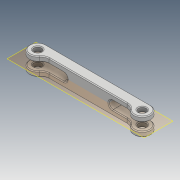
# Autodesk Inventor part: bar_act_ab
Saved by Autodesk Inventor 2018 (Build 220112000, 112)
## iProperties
Created: 2019-01-31
Part Number: bar_act_ab
Material: Generic
Document SubType Name: Modeling
Designer: Tsche
Density: 1 g/cm^3
Appearance: Default
Author: Tsche
Autodesk Inventor part; units mm, degrees
ref_plane "YZ Plane" through (0, 0, 0) normal (1, 0, 0) x (0, 1, 0)
ref_plane "XZ Plane" through (0, 0, 0) normal (0, 1, 0) x (-1, 0, 0)
ref_plane "XY Plane" through (0, 0, 0) normal (0, 0, 1) x (1, 0, 0)
sketch "Sketch1" plane through (0, 0, 0) normal (0, 0, 1) x (1, 0, 0)
  circle A0 centre (20.2406, 0) radius 1.4625
  line L0 (20.2406, 3.25) -> (-2.6872, 3.25)
  line L1 (-446494.9011, 0) -> (446494.9011, 0) construction
  line L2 (0, -0.75) -> (15.1171, -0.75)
  arc A1 (17.6789, -2) -> (20.2406, 3.25) centre (20.2406, 0) ccw
  arc A2 (17.6789, -2) -> (15.1171, -0.75) centre (15.1171, -4) ccw
  line L3 (0, -446500.8256) -> (0, 446500.0254) construction
  circle A3 centre (-20.2406, 0) radius 1.4625
  line L4 (-20.2406, 3.25) -> (-2.6872, 3.25)
  line L5 (446494.9011, 0) -> (-446494.9011, 0) construction
  line L6 (0, -0.75) -> (-15.1171, -0.75)
  arc A4 (-20.2406, 3.25) -> (-17.6789, -2) centre (-20.2406, 0) ccw
  arc A5 (-15.1171, -0.75) -> (-17.6789, -2) centre (-15.1171, -4) ccw
  point P0 (0, 0)
  dimension "d0" = 4
  dimension "d1" = 3.25
  dimension "d2" = 3.25
  dimension "d3" = 2.925
  dimension "d4" = 40.4813
  constraints: 10 end point, 8 horizontal alignment, 8 point on circle, 6 centre point, 3 equal radius, 3 tangent, 2 coincident, 2 horizontal, 2 point on line, 2 other
  measures "d0" distance between parallel lines of L0 L2
  measures "d1" radius of A1
  measures "d2" radius of A2
  measures "d3" diameter of A0
  measures "d4" distance of A0.centre A3.centre
extrude "Extrusion1" add sketch "Sketch1" along normal blind 7
ref_plane "Work Plane1" through (0, 0, 3.5) normal (0, 0, 1) x (1, 0, 0)
sketch "Sketch2" plane through (-20.2406, 3.25, 0) normal (0, 1, 0) x (1, 0, 0)
  line L0 (53.1275, -3.5) -> (-12.6463, -3.5) construction
  line L1 (43.7313, 0) -> (43.7313, -7) construction
  line L2 (43.7313, -1.9625) -> (29.7613, -1.9625)
  line L3 (43.7313, -5.0375) -> (29.7613, -5.0375)
  arc A0 (29.7613, -1.9625) -> (29.7613, -5.0375) centre (29.7613, -3.5) ccw
  line L4 (43.7313, -1.9625) -> (43.7313, -5.0375)
  line L5 (20.2406, 1.4) -> (20.2406, -8.4) construction
  line L6 (-3.25, -1.9625) -> (10.72, -1.9625)
  line L7 (-3.25, -5.0375) -> (10.72, -5.0375)
  arc A1 (10.72, -5.0375) -> (10.72, -1.9625) centre (10.72, -3.5) ccw
  line L8 (-3.25, -1.9625) -> (-3.25, -5.0375)
  point P0 (20.2406, 0)
  dimension "d7" = 3.075
  dimension "d9" = 13.97
  constraints: 12 end point, 7 symmetric about line, 4 point on circle, 2 centre point, 1 collinear, 1 perpendicular, 1 point on line, 1 tangent, 1 other
  measures "d7" distance between parallel lines of L2 L3
  measures "d9" distance from line of L1 A0.centre
extrude "Extrusion2" cut sketch "Sketch2" against normal through all
chamfer "Chamfer1" distance 0.3 angle 45 26 edges at (0, -0.75, 7) (16.5424, -1.0792, 7) (23.1615, -1.4252, 7) (0, 3.25, 7) (-23.1615, -1.4252, 7) (-16.5424, -1.0792, 7) (0, -0.75, 0) (16.5424, -1.0792, 0) (23.1615, -1.4252, 0) (0, 3.25, 0) (-23.1615, -1.4252, 0) (-16.5424, -1.0792, 0) (7.9831, -0.75, 3.5) (12.3189, -0.75, 5.0375) (16.5424, -1.0792, 5.0375) (23.1615, -1.4252, 5.0375) (23.1615, -1.4252, 1.9625) (16.5424, -1.0792, 1.9625) (12.3189, -0.75, 1.9625) (-16.5424, -1.0792, 1.9625) (-23.1615, -1.4252, 1.9625) (-14.8806, 3.25, 1.9625) (-7.9831, 3.25, 3.5) (-14.8806, 3.25, 5.0375) (-23.1615, -1.4252, 5.0375) (-16.5424, -1.0792, 5.0375)
fillet "Fillet1" radius 0.3 8 edges at (-21.7031, 0, 0) (-21.7031, 0, 1.9625) (-21.7031, 0, 5.0375) (-21.7031, 0, 7) (18.7781, 0, 5.0375) (18.7781, 0, 7) (18.7781, 0, 1.9625) (18.7781, 0, 0)
equation "\"d0\" = bar_thickness"
equation "\"d1\" = 0.5 * bar_diameter"
equation "\"d2\" = 0.5 * bar_diameter"
equation "\"d3\" = bore_press"
equation "\"d4\" = bar_act_length_ab"
equation "\"d5\" = bar_width"
equation "\"d7\" = hinge_thickness + finger_link_clearence"
equation "\"d10\" = hinge_thickness"
equation "\"d12\" = champfer"
equation "\"bar_length_bc\" = finger_part_B_length"
equation "\"hinge_thickness\" = 3"
equation "\"bar_diameter\" = 6.5"
equation "\"bore_clearance\" = 3.025"
equation "\"finger_width\" = 25"
equation "\"finger_thickness\" = 8"
equation "\"finger_part_A_length\" = 42.8625"
equation "\"finger_part_B_length\" = 28.575"
equation "\"finger_link_width\" = 3.5"
equation "\"finger_link_clearence\" = 0.075"
equation "\"tol\" = 0.5 * finger_link_clearence"
equation "\"link_tol\" = 0.254"
equation "\"bore_press\" = 2.925"
equation "\"bar_thickness\" = 4"
equation "\"hinge_dist_sym_plane\" = 4"
equation "\"hinge_act_length_c\" = 7.62"
equation "\"hinge_act_length_bc\" = 16.66875"
equation "\"hinge_act_length_ab\" = 11.049"
equation "\"hinge_act_length_a\" = 21.43125"
equation "\"hinge_guid_length_c\" = 9.525"
equation "\"hinge_guid_length_bc\" = 9.525"
equation "\"hinge_guid_length_ab\" = 17.145"
equation "\"hinge_guid_length_a\" = 17.145"
equation "\"bar_act_length_ab\" = 40.48125"
equation "\"bar_guid_length_ab\" = 43.275"
equation "\"bar_width\" = 7"
equation "\"champfer\" = 0.3"
equation "\"fillet\" = 0.4"
equation "\"dist_finger_BC\" = 56.5"
equation "\"gear_diameter\" = 14"
equation "\"hinge_point\" = 15"
body "Solid1"
